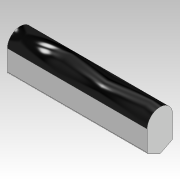
# Autodesk Inventor part: ApexSeal
Saved by Autodesk Inventor 2020 (Build 240168000, 168)
## iProperties
Created: 2021-10-16
Part Number: ApexSeal
Material: Generic
Document SubType Name: Modeling
Designer: DDeGo
Density: 1 g/cm^3
Appearance: Default
Author: DDeGo
Autodesk Inventor part; units mm, degrees
ref_plane "YZ Plane" through (0, 0, 0) normal (1, 0, 0) x (0, 1, 0)
ref_plane "XZ Plane" through (0, 0, 0) normal (0, 1, 0) x (-1, 0, 0)
ref_plane "XY Plane" through (0, 0, 0) normal (0, 0, 1) x (1, 0, 0)
sketch "Sketch1" plane through (0, 0, 0) normal (1, 0, 0) x (0, 1, 0)
  line L0 (-0.85, 1) -> (0.85, 1)
  line L1 (0.85, -1) -> (-0.85, -1)
  line L2 (-0.85, -1) -> (-0.85, 1) construction
  line L3 (-0.85, 1) -> (0.85, -1) construction
  line L4 (0.85, 1) -> (-0.85, -1) construction
  arc A0 (0.85, 1) -> (0.85, -1) centre (0.85, 0) ccw
  line L5 (-0.85, 1) -> (-1.35, 0)
  line L6 (-1.35, 0) -> (-0.85, -1)
  point P0 (0, 0)
  dimension "d0" = 2
  dimension "d1" = 1.7
  dimension "d9" = 2.2
  constraints: 14 end point, 2 midpoint, 2 point on circle, 2 tangent, 1 centre point, 1 equal length, 1 horizontal, 1 parallel, 1 perpendicular
  measures "d0" distance between parallel lines of L1 L0
  measures "d1" distance of L1.start L1.end
  measures "d9" horizontal distance of L1.start L5.end
extrude "Extrusion1" add sketch "Sketch1" along normal mid plane 11
fillet "Fillet1" radius 0.05 2 edges at (0, 0.85, 1) (0, 0.85, -1)
fillet "Fillet1" radius 0.15 3 edges at (0, -0.85, -1) (0, -0.85, 1) (0, -1.35, 0)
sketch "Sketch2" plane through (0, 0, 0) normal (1, 0, 0) x (0, 1, 0)
  arc A0 (0.85, 1) -> (0.85, -1) centre (0.85, 0) ccw projected
  circle A1 centre (0.85, 0) radius 1
  line L0 (-0.7573, 1) -> (0.4028, 1) projected
  line L1 (0.4028, 1) -> (0.85, 1)
  line L2 (0.85, 1) -> (0.85, -1)
  line L3 (-0.7573, -1) -> (0.4028, -1) projected
  line L4 (0.85, -1) -> (0.4028, -1)
  arc A2 (-1.3165, 0.0671) -> (-1.3165, -0.0671) centre (-1.1823, 0) ccw projected
  line L5 (-1.3165, -0.0671) -> (-0.8915, -0.9171) projected
  arc A3 (-0.8915, -0.9171) -> (-0.7573, -1) centre (-0.7573, -0.85) ccw projected
  line L6 (-0.7573, -1) -> (0.4028, -1) projected
  arc A4 (0.4028, -1) -> (0.4241, -0.9048) centre (0.4028, -0.95) ccw projected
  arc A5 (0.4241, 0.9048) -> (0.4241, -0.9048) centre (0.85, 0) ccw projected
  arc A6 (0.4241, 0.9048) -> (0.4028, 1) centre (0.4028, 0.95) ccw projected
  line L7 (0.4028, 1) -> (-0.7573, 1) projected
  arc A7 (-0.7573, 1) -> (-0.8915, 0.9171) centre (-0.7573, 0.85) ccw projected
  line L8 (-0.8915, 0.9171) -> (-1.3165, 0.0671) projected
  point P0 (0, 0)
  point P1 (0.85, 1)
  point P2 (0.4241, 0.9048)
  point P3 (0.4241, -0.9048)
  constraints: 6 end point, 2 collinear, 1 coincident, 1 horizontal, 1 perpendicular, 1 tangent, 3 other
extrude "graphite" add sketch "Sketch2" along normal mid plane 11 contours L2 A0 | A0 A6 L1 | A1 L2 | L4 A4 A0
body "Solid1"
